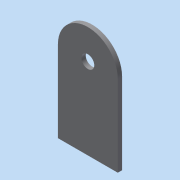
# Autodesk Inventor part: 草圖檔
Saved by Autodesk Inventor 2013 (Build 170138000, 138)
## iProperties
Created: 2015-10-26
Part Number: 草圖檔
Document SubType Name: Modeling
Designer: user
Density: 1 g/cm^3
Material: 一般
Author: user
Autodesk Inventor part; units mm, degrees
ref_plane "YZ Plane" through (0, 0, 0) normal (1, 0, 0) x (0, 1, 0)
ref_plane "XZ Plane" through (0, 0, 0) normal (0, 1, 0) x (-1, 0, 0)
ref_plane "XY Plane" through (0, 0, 0) normal (0, 0, 1) x (1, 0, 0)
sketch "草圖2" plane through (0, 0, 0) normal (0, 1, 0) x (-1, 0, 0)
  line L0 (0, 0) -> (25, 0) construction
  line L1 (0, 0) -> (0, 21.0714) construction
  line L2 (-14, 0) -> (14, 0)
  line L3 (14, 0) -> (14, 38)
  line L4 (-14, 38) -> (-14, 0)
  arc A0 (14, 38) -> (-14, 38) centre (0, 38) ccw
  circle A1 centre (0, 38) radius 3
  dimension "d1" = 28
  dimension "d3" = 38
  dimension "d4" = 6
  dimension "d5" = 52
  constraints: 10 end point, 2 centre point, 2 horizontal, 2 perpendicular, 2 point on circle, 2 tangent, 1 coincident, 1 midpoint, 1 parallel, 1 other
  measures "d1" distance between parallel lines of L3 L4
  measures "d3" distance from line of L2 A0.centre
  measures "d4" diameter of A1
extrude "擠出1" add sketch "草圖2" along normal mid plane 2
